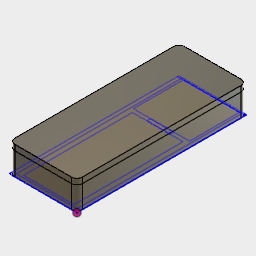
Digibtooth (Autodesk Fusion 360 design; units mm, degrees)
Autodesk Fusion 360 part; units mm, degrees
sketch "Sketch1" plane through (0, 0, 0) normal (0, 1, 0) x (1, 0, 0)
  line L0 (0, 0) -> (-24, 0)
  line L1 (-24, 0) -> (-24, 59.75)
  line L2 (-24, 59.75) -> (0, 59.75)
  line L3 (0, 59.75) -> (0, 0)
  line L4 (-3, 40.6927) -> (-21, 40.6927)
  line L5 (-21, 40.6927) -> (-21, 2)
  line L6 (-21, 2) -> (-3, 2)
  line L7 (-3, 2) -> (-3, 40.6927)
  line L8 (-22, 59.75) -> (-2, 59.75)
  line L9 (-2, 59.75) -> (-2, 42)
  line L10 (-2, 42) -> (-22, 42)
  line L11 (-22, 42) -> (-22, 59.75)
  line L12 (-22.75, 1.25) -> (-1.25, 1.25)
  line L13 (-1.25, 1.25) -> (-1.25, 59.75)
  line L14 (-1.25, 59.75) -> (-22.75, 59.75)
  line L15 (-22.75, 59.75) -> (-22.75, 1.25)
  line L16 (-15.8885, 42) -> (-7.5321, 42)
  line L17 (-7.5321, 42) -> (-7.5321, 40.6927)
  line L18 (-7.5321, 40.6927) -> (-15.8885, 40.6927)
  line L19 (-15.8885, 40.6927) -> (-15.8885, 42)
  line L20 (0, 59.75) -> (-5.5359, 59.75)
  line L21 (-5.5359, 59.75) -> (-5.5359, 60.25)
  line L22 (-5.5359, 60.25) -> (0, 60.25)
  line L23 (0, 60.25) -> (0, 59.75)
  line L24 (-24, 59.75) -> (-18.4999, 59.75)
  line L25 (-18.4999, 59.75) -> (-18.4999, 60.25)
  line L26 (-18.4999, 60.25) -> (-24, 60.25)
  line L27 (-24, 60.25) -> (-24, 59.75)
  line L28 (-18.4999, 59.75) -> (-5.5359, 59.75)
  line L29 (-5.5359, 59.75) -> (-5.5359, 60.25)
  line L30 (-5.5359, 60.25) -> (-18.4999, 60.25)
  line L31 (-18.4999, 60.25) -> (-18.4999, 59.75)
  dimension "d17" = 0.5
  dimension "d19" = 0.5
  constraint horizontal L0
  constraint vertical L1
  constraint horizontal L2
  constraint vertical L3
  constraint horizontal L4
  constraint vertical L5
  constraint horizontal L6
  constraint vertical L7
  constraint horizontal L8
  constraint vertical L9
  constraint horizontal L10
  constraint vertical L11
  constraint horizontal L12
  constraint vertical L13
  constraint horizontal L14
  constraint vertical L15
  constraint coincident L2
  constraint horizontal L16
  constraint vertical L17
  constraint horizontal L18
  constraint vertical L19
  constraint coincident L4
  constraint coincident L10
  constraint horizontal L20
  constraint vertical L21
  constraint horizontal L22
  constraint vertical L23
  constraint horizontal L24
  constraint vertical L25
  constraint horizontal L26
  constraint vertical L27
extrude "Extrude3" add sketch "Sketch1" along normal blind 8 contours L0 L1 L2 L3 L12 L13 L15 L20 L24 makes body 1
extrude "Extrude4" add sketch "Sketch1" along normal blind 6.5 contours L2 L4 L5 L6 L7 L9 L10 L11 L12 L13 L14 L15 L17 L19 L20 L24 bodies 1
extrude "Extrude5" add sketch "Sketch1" along normal blind 2 contours L2 L8 L9 L10 L11 L14 L16 L20 L24 L28 | L4 L10 L16 L17 L18 L19 | L4 L5 L6 L7 L18 bodies 1
extrude "Extrude9" add sketch "Sketch1" along normal blind 8 contours L2 L8 L14 L20 L21 L22 L23 L29 | L2 L8 L14 L24 L25 L26 L27 L31 bodies 1
extrude "Extrude10" add sketch "Sketch1" along normal blind 2 contours L2 L8 L14 L21 L25 L28 L29 L30 L31 bodies 1
extrude "Extrude11" add sketch "Sketch1" along normal blind 2 separate body makes body 2
extrude "Extrude12" add sketch "Sketch1" along normal blind 3.5 contours L2 L4 L5 L6 L7 L9 L10 L11 L12 L13 L14 L15 L17 L19 L20 L24 | L2 L8 L9 L10 L11 L14 L16 L20 L24 L28 | L4 L10 L16 L17 L18 L19 | L4 L5 L6 L7 L18 bodies 2
extrude "Extrude13" add sketch "Sketch1" along normal blind 3.5 contours L2 L8 L14 L21 L25 L28 L29 L30 L31 bodies 2
move_face "OffsetFaces2" offset -1.75 1 faces at (-21.3333, 2.5, -59.75) on bodies 2
move_face "OffsetFaces3" offset -1.75 1 faces at (-4.1073, 2.5, -59.75) on bodies 2
move_body "MoveBody6" bodies 2 to x (-1, 0, 0) y (0, -1, 0) z (0, 0, 1) at (-48, 0, 0)
move_body "MoveBody7" bodies 2 to x (1, 0, 0) y (0, 1, 0) z (0, 0, 1) at (24, 10, 0)
fillet "Fillet1" radius 2 8 edges at (0, 4, -60.25) (-24, 4, -60.25) (-24, 4, 0) (0, 4, 0) (0, 9, -60.25) (-24, 9, -60.25) (-24, 9, 0) (0, 9, 0) on bodies 1 2
